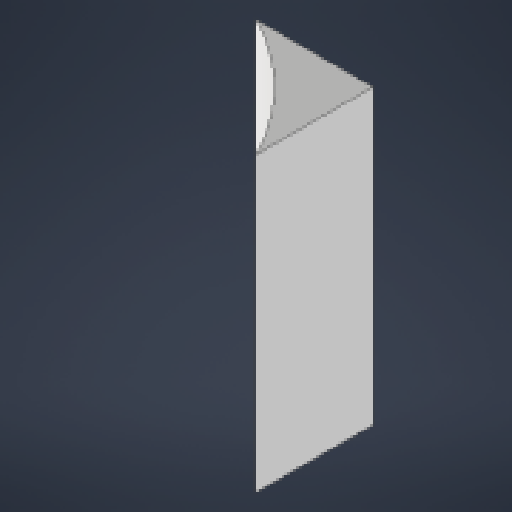
# Autodesk Inventor part: coral_guide
Saved by Autodesk Inventor 2024.3 (Build 283343010, 343A)
## iProperties
Created: 2025-03-08
Part Number: coral_guide
Material: Generic
Document SubType Name: Modeling
Designer: Owen L
Density: 1 g/cm^3
Appearance: Default
Author: Owen L
Autodesk Inventor part; units mm, degrees
ref_plane "YZ Plane" through (0, 0, 0) normal (1, 0, 0) x (0, 1, 0)
ref_plane "XZ Plane" through (0, 0, 0) normal (0, 1, 0) x (-1, 0, 0)
ref_plane "XY Plane" through (0, 0, 0) normal (0, 0, 1) x (1, 0, 0)
sketch "Sketch1" plane through (0, 0, 0) normal (1, 0, 0) x (0, 0, 1)
  line L0 (12.7, 69.85) -> (-12.7, 69.85)
  line L1 (-12.7, 69.85) -> (-12.7, -69.85)
  line L2 (-12.7, -69.85) -> (12.7, -69.85)
  line L3 (12.7, -69.85) -> (12.7, 69.85)
  line L4 (12.7, 69.85) -> (-12.7, -69.85) construction
  line L5 (-12.7, 69.85) -> (12.7, -69.85) construction
  point P0 (0, 0)
  dimension "d3" = 25.4
  dimension "d4" = 139.7
  constraints: 12 end point, 2 midpoint, 2 parallel, 1 horizontal, 1 perpendicular
  measures "d3" distance of L2.end L1.end
  measures "d4" distance of L1.end L0.end
extrude "Extrusion1" add sketch "Sketch1" along normal blind 12.7
sketch "Sketch2" plane through (0, 69.85, 12.7) normal (0, 1, 0) x (1, 0, 0)
  circle A0 centre (-34.819, -31.75) radius 57.15
  line L0 (0, 25.4) -> (12.7, 25.4) projected
  point P0 (0, 12.7)
  point P1 (12.7, 0)
  dimension "d7" = 114.3
  constraints: 1 horizontal, 3 other
extrude "Extrusion2" cut sketch "Sketch2" against normal through all
chamfer "Chamfer1" distance 17.1747 distance2 50.8 1 edges at (6.9052, 69.85, 5.3961) measured on face at (7.2703, 69.85, 5.0544)
fillet "Fillet1" radius 76.2 1 edges at (6.9052, 19.05, 5.3961)
sketch "Sketch3" plane through (12.8807, -69.1617, -12.7) normal (0, 0, -1) x (-1, 0, 0)
  line L0 (6.5307, 12.0117) -> (6.5307, 113.6117) construction
  line L1 (6.5307, 12.0117) -> (6.5307, 62.8117) construction
  line L2 (6.5307, 62.8117) -> (6.5307, 113.6117) construction
  line L3 (12.8807, -0.6883) -> (0.1807, -0.6883) projected
  line L4 (0.1807, -0.6883) -> (0.1807, 139.0117) projected
  point P0 (6.5307, 37.4117)
  point P1 (6.5307, 88.2117)
  dimension "d23" = 12.7
  dimension "d24" = 6.35
  dimension "d25" = 101.6
  constraints: 6 end point, 3 midpoint, 2 coincident, 1 collinear, 1 vertical
  measures "d23" distance from line of L3 L0.start
  measures "d24" distance from line of L4 L0.start
  measures "d25" distance of L0.start L0.end
hole "Hole1" at (6.35, -57.15, -12.7) at (6.35, -6.35, -12.7) at (6.35, -31.75, -12.7) at (6.35, 19.05, -12.7) direction (0, 0, 1) diameter 5.639 depth 5.969 tip angle 118
body "Solid1"
